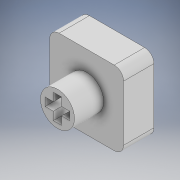
# Autodesk Inventor part: IPC 3 key
Saved by Autodesk Inventor 2022 (Build 260153000, 153)
## iProperties
Created: 2021-12-31
Part Number: IPC 3 key
Material: Generic
Document SubType Name: Modeling
Designer: solor
Density: 1 g/cm^3
Appearance: Default
Author: solor
Autodesk Inventor part; units mm, degrees
ref_plane "YZ Plane" through (0, 0, 0) normal (1, 0, 0) x (0, 1, 0)
ref_plane "XZ Plane" through (0, 0, 0) normal (0, 1, 0) x (-1, 0, 0)
sketch "Sketch1" plane through (0, 0, 0) normal (0, 0, 1) x (1, 0, 0)
  line L0 (14.6962, 12.74) -> (14.6962, 0) construction
  line L1 (10.61, 12.2) -> (1.53, 12.2)
  arc A0 (1.53, 12.2) -> (0, 10.67) centre (1.53, 10.67) ccw
  line L2 (0, 10.67) -> (0, 1.53)
  arc A1 (0, 1.53) -> (1.53, 0) centre (1.53, 1.53) ccw
  line L3 (1.53, 0) -> (10.61, 0)
  arc A2 (10.61, 0) -> (12.14, 1.53) centre (10.61, 1.53) ccw
  arc A3 (12.14, 10.67) -> (10.61, 12.2) centre (10.61, 10.67) ccw
  line L4 (12.14, 10.67) -> (12.14, 1.53)
  point P0 (0, 0)
  point P1 (0, 0)
  dimension "d10" = 12.74
  constraints: 10 end point, 8 point on circle, 4 centre point, 2 vertical, 1 point on line
  measures "d10" distance of L0.start L0.end
ref_plane "Work Plane1" through (0, 0, 5) normal (0, 0, 1) x (1, 0, 0)
sketch "Sketch2" plane through (0, 0, 5) normal (0, 0, 1) x (1, 0, 0)
  line L0 (10.88, 12.74) -> (1.8, 12.74) projected
  line L1 (10.88, 12.74) -> (1.8, 12.74) projected
  arc A0 (1.8, 12.74) -> (0, 10.94) centre (1.8, 10.94) ccw projected
  line L2 (0, 10.94) -> (0, 1.8) projected
  arc A1 (0, 1.8) -> (1.8, 0) centre (1.8, 1.8) ccw projected
  line L3 (1.8, 0) -> (10.88, 0) projected
  arc A2 (10.88, 0) -> (12.68, 1.8) centre (10.88, 1.8) ccw projected
  line L4 (12.68, 1.8) -> (12.68, 10.94) projected
  arc A3 (12.68, 10.94) -> (10.88, 12.74) centre (10.88, 10.94) ccw projected
  circle A4 centre (6.34, 6.37) radius 2.8
  line L5 (5.665, 8.395) -> (7.015, 8.395)
  line L6 (7.015, 4.345) -> (5.665, 4.345)
  line L7 (5.665, 4.345) -> (7.015, 8.395) construction
  line L8 (5.665, 8.395) -> (7.015, 4.345) construction
  line L9 (8.365, 5.695) -> (8.365, 7.045)
  line L10 (4.315, 7.045) -> (4.315, 5.695)
  line L11 (4.315, 5.695) -> (8.365, 7.045) construction
  line L12 (8.365, 5.695) -> (4.315, 7.045) construction
  line L13 (4.315, 5.695) -> (5.665, 5.695)
  line L14 (7.015, 5.695) -> (8.365, 5.695)
  line L15 (5.665, 4.345) -> (5.665, 5.695)
  line L16 (5.665, 7.045) -> (5.665, 8.395)
  line L17 (8.365, 7.045) -> (7.015, 7.045)
  line L18 (5.665, 7.045) -> (4.315, 7.045)
  line L19 (7.015, 8.395) -> (7.015, 7.045)
  line L20 (7.015, 5.695) -> (7.015, 4.345)
  point P0 (0, 0)
  dimension "d3" = 5.6
  dimension "d4" = 4.05
  dimension "d5" = 1.35
  dimension "d6" = 4.05
  dimension "d7" = 1.35
  constraints: 32 end point, 10 parallel, 8 perpendicular, 4 midpoint, 2 vertical, 1 centre point
  measures "d3" diameter of A4
  measures "d4" distance of L6.end L5.start
  measures "d5" distance of L5.start L5.end
  measures "d6" distance of L10.end L9.start
  measures "d7" distance of L9.end L9.start
extrude "Extrusion3" add sketch "Sketch1" along normal blind 5
sketch "Sketch3" plane through (0, 0, 5) normal (0, 0, 1) x (1, 0, 0)
  line L0 (10.61, 12.47) -> (1.53, 12.47)
  line L1 (10.61, 12.47) -> (1.53, 12.47)
  arc A0 (1.53, 12.47) -> (-0.27, 10.67) centre (1.53, 10.67) ccw
  line L2 (-0.27, 10.67) -> (-0.27, 1.53)
  arc A1 (-0.27, 1.53) -> (1.53, -0.27) centre (1.53, 1.53) ccw
  line L3 (1.53, -0.27) -> (10.61, -0.27)
  arc A2 (10.61, -0.27) -> (12.41, 1.53) centre (10.61, 1.53) ccw
  line L4 (12.41, 1.53) -> (12.41, 10.67)
  arc A3 (12.41, 10.67) -> (10.61, 12.47) centre (10.61, 10.67) ccw
  circle A4 centre (6.07, 6.1) radius 2.8
  line L5 (5.395, 8.125) -> (6.745, 8.125)
  line L6 (6.745, 4.075) -> (5.395, 4.075)
  line L7 (5.395, 4.075) -> (6.745, 8.125) construction
  line L8 (5.395, 8.125) -> (6.745, 4.075) construction
  line L9 (8.095, 5.425) -> (8.095, 6.775)
  line L10 (4.045, 6.775) -> (4.045, 5.425)
  line L11 (4.045, 5.425) -> (8.095, 6.775) construction
  line L12 (8.095, 5.425) -> (4.045, 6.775) construction
  line L13 (4.045, 5.425) -> (5.395, 5.425)
  line L14 (6.745, 5.425) -> (8.095, 5.425)
  line L15 (5.395, 4.075) -> (5.395, 5.425)
  line L16 (5.395, 6.775) -> (5.395, 8.125)
  line L17 (8.095, 6.775) -> (6.745, 6.775)
  line L18 (5.395, 6.775) -> (4.045, 6.775)
  line L19 (6.745, 8.125) -> (6.745, 6.775)
  line L20 (6.745, 5.425) -> (6.745, 4.075)
  line L21 (10.61, 12.2) -> (1.53, 12.2) projected
  line L22 (0, 10.67) -> (0, 1.53) projected
  point P0 (0, 0)
  point P1 (-0.27, -0.27)
  point P2 (6.07, 12.2)
  point P3 (0, 6.1)
  point P4 (6.07, 6.1)
  dimension "d14" = 5.6
  dimension "d15" = 4.05
  dimension "d16" = 1.35
  dimension "d17" = 4.05
  dimension "d18" = 1.35
  constraints: 42 end point, 10 parallel, 8 perpendicular, 8 point on circle, 6 midpoint, 5 centre point, 2 vertical
  measures "d14" diameter of A4
  measures "d15" distance of L6.end L5.start
  measures "d16" distance of L5.start L5.end
  measures "d17" distance of L10.end L9.start
  measures "d18" distance of L9.end L9.start
extrude "Extrusion4" add sketch "Sketch3" along normal blind 4.8 contours A4
sketch "Sketch4" plane through (0, 0, 0) normal (0, 0, -1) x (-1, 0, 0)
  line L0 (-13.9436, 0) -> (-13.9436, 2.266)
  line L1 (-15.5559, 0) -> (-15.5559, 6.84)
  line L2 (-1.53, 0) -> (-10.61, 0) projected
  line L3 (-7.4059, 5.4445) -> (-4.7341, 5.4445) construction
  line L4 (-4.7341, 5.4445) -> (-4.7341, 2.266) construction
  line L5 (-4.7341, 2.266) -> (-7.4059, 2.266) construction
  line L6 (-7.4059, 2.266) -> (-7.4059, 5.4445) construction
  spline S0 degree 2 poles (-4.9318, 3.2547) (-4.9318, 3.0297) (-5.0974, 2.6615) (-5.2581, 2.5329) knots 0 0 0 1 2 2 2
  spline S1 degree 2 poles (-5.2581, 2.5329) (-5.4187, 2.4044) (-5.8562, 2.266) (-6.1701, 2.266) knots 0 0 0 1 2 2 2
  spline S2 degree 2 poles (-6.1701, 2.266) (-6.526, 2.266) (-7.0352, 2.3846) (-7.1958, 2.4588) knots 0 0 0 1 2 2 2
  line L7 (-7.1958, 2.4588) -> (-7.1958, 3.1212)
  line L8 (-7.1958, 3.1212) -> (-7.1217, 3.1212)
  spline S3 degree 2 poles (-7.1217, 3.1212) (-6.9536, 3.0149) (-6.5013, 2.8567) (-6.3135, 2.8567) knots 0 0 0 1 2 2 2
  spline S4 degree 2 poles (-6.3135, 2.8567) (-6.2022, 2.8567) (-5.9427, 2.8963) (-5.8537, 2.9605) knots 0 0 0 1 2 2 2
  spline S5 degree 2 poles (-5.8537, 2.9605) (-5.7845, 3.0124) (-5.7005, 3.1632) (-5.7005, 3.2991) knots 0 0 0 1 2 2 2
  spline S6 degree 2 poles (-5.7005, 3.2991) (-5.7005, 3.4351) (-5.8191, 3.5809) (-5.918, 3.6155) knots 0 0 0 1 2 2 2
  spline S7 degree 2 poles (-5.918, 3.6155) (-6.0169, 3.6501) (-6.2912, 3.6575) (-6.3975, 3.6575) knots 0 0 0 1 2 2 2
  line L9 (-6.3975, 3.6575) -> (-6.5285, 3.6575)
  line L10 (-6.5285, 3.6575) -> (-6.5285, 4.1939)
  line L11 (-6.5285, 4.1939) -> (-6.4074, 4.1939)
  spline S8 degree 2 poles (-6.4074, 4.1939) (-6.269, 4.1939) (-6.0342, 4.2186) (-5.9526, 4.2557) knots 0 0 0 1 2 2 2
  spline S9 degree 2 poles (-5.9526, 4.2557) (-5.871, 4.2952) (-5.7796, 4.4336) (-5.7796, 4.5523) knots 0 0 0 1 2 2 2
  spline S10 degree 2 poles (-5.7796, 4.5523) (-5.7796, 4.6462) (-5.8661, 4.7624) (-5.9279, 4.7945) knots 0 0 0 1 2 2 2
  spline S11 degree 2 poles (-5.9279, 4.7945) (-6.002, 4.8316) (-6.1998, 4.8563) (-6.269, 4.8563) knots 0 0 0 1 2 2 2
  spline S12 degree 2 poles (-6.269, 4.8563) (-6.3802, 4.8563) (-6.615, 4.8044) (-6.7237, 4.7624) knots 0 0 0 1 2 2 2
  spline S13 degree 2 poles (-6.7237, 4.7624) (-6.8103, 4.7302) (-6.9981, 4.6264) (-7.0426, 4.5992) knots 0 0 0 1 2 2 2
  line L12 (-7.0426, 4.5992) -> (-7.1069, 4.5992)
  line L13 (-7.1069, 4.5992) -> (-7.1069, 5.2517)
  spline S14 degree 2 poles (-7.1069, 5.2517) (-6.9487, 5.3185) (-6.4148, 5.4445) (-6.1355, 5.4445) knots 0 0 0 1 2 2 2
  spline S15 degree 2 poles (-6.1355, 5.4445) (-5.8636, 5.4445) (-5.4632, 5.3506) (-5.3223, 5.2592) knots 0 0 0 1 2 2 2
  spline S16 degree 2 poles (-5.3223, 5.2592) (-5.1666, 5.1628) (-5.0109, 4.8662) (-5.0109, 4.6808) knots 0 0 0 1 2 2 2
  spline S17 degree 2 poles (-5.0109, 4.6808) (-5.0109, 4.4188) (-5.3124, 4.0283) (-5.5596, 3.9714) knots 0 0 0 1 2 2 2
  line L14 (-5.5596, 3.9714) -> (-5.5596, 3.9418)
  spline S18 degree 2 poles (-5.5596, 3.9418) (-5.4509, 3.9269) (-5.2432, 3.8478) (-5.1444, 3.7589) knots 0 0 0 1 2 2 2
  spline S19 degree 2 poles (-5.1444, 3.7589) (-5.0529, 3.6798) (-4.9318, 3.4277) (-4.9318, 3.2547) knots 0 0 0 1 2 2 2
  point P0 (0, 0)
  point P1 (-6.07, 0)
  point P2 (-6.07, 2.266)
  point P3 (-6.07, 6.84)
  point P4 (-6.07, 2.266)
  dimension "d21" = 2.266
  dimension "d22" = 6.84
  constraints: 4 end point, 2 midpoint, 2 vertical, 2 other
  measures "d21" distance of L0.start L0.end
  measures "d22" distance of L1.start L1.end
extrude "Extrusion5" add sketch "Sketch4" along normal blind 0.9
body "Solid2"
